Autodesk Fusion 360 part; units mm, degrees
note: some values were not read from the file. Chosen so that the rebuilt part matches the saved one: which face or edge a step refers to. Set by a fixed rule: which sketch regions a step uses.
(part 2 of 2)
extrude "Extrude26" cut sketch "Enclosure_upper" along normal blind 2 from surface at -3 contours L33 L34 L35 L36 bodies 2
extrude "Extrude27" add sketch "Enclosure_main" along normal blind 5 contours A4 | A6 | A8 | A9 | A12 | A13 | A14 | A18 | A19 | A22 | A23 bodies 1
sketch "bkac_plate" plane through (0, 0, -3) normal (0, 0, -1) x (-1, 0, 0)
  line L0 (-20, 60) -> (-210, 60)
  line L1 (-210, 60) -> (-210, -3)
  line L2 (-210, -3) -> (-20, -3)
  line L3 (-20, -3) -> (-20, 60)
  line L4 (-56.5, 6.25) -> (-39.5, 6.25)
  line L5 (-39.5, 6.25) -> (-39.5, 1.25)
  line L6 (-39.5, 1.25) -> (-56.5, 1.25)
  line L7 (-56.5, 1.25) -> (-56.5, 6.25)
  line L8 (3, -3) -> (3, 60)
  line L9 (-133.8, 16.5) -> (-117.5, 16.5)
  line L10 (-117.5, 16.5) -> (-117.5, 3)
  line L11 (-117.5, 3) -> (-133.8, 3)
  line L12 (-133.8, 3) -> (-133.8, 16.5)
  line L13 (0, 0) -> (-230, 0)
  circle A0 centre (-139.55, 11) radius 2
  circle A1 centre (-111.75, 11) radius 2
  circle A2 centre (-198.8, 12) radius 8
  circle A3 centre (-198.8, 37) radius 6
  line L14 (-206.05, 19.25) -> (-191.55, 19.25)
  line L15 (-191.55, 19.25) -> (-191.55, 4.75)
  line L16 (-191.55, 4.75) -> (-206.05, 4.75)
  line L17 (-206.05, 4.75) -> (-206.05, 19.25)
  line L18 (-206.05, 12) -> (-191.55, 12) construction
  line L19 (-198.8, 19.25) -> (-198.8, 4.75) construction
  line L20 (-204.25, 42.45) -> (-193.35, 42.45)
  line L21 (-193.35, 42.45) -> (-193.35, 31.55)
  line L22 (-193.35, 31.55) -> (-204.25, 31.55)
  line L23 (-204.25, 31.55) -> (-204.25, 42.45)
  line L24 (-204.25, 37) -> (-193.35, 37) construction
  line L25 (-198.8, 42.45) -> (-198.8, 31.55) construction
  circle A4 centre (-183.8, 25) radius 3.25
  point P0 (0, -20)
  dimension "d451" = 17
  dimension "d452" = 5
  dimension "d453" = 51
  dimension "d454" = 4.25
  dimension "d459" = 16.3
  dimension "d460" = 13.5
  dimension "d461" = 3
  dimension "d462" = 4
  dimension "d463" = 5.75
  dimension "d464" = 4
  dimension "d465" = 5.75
  dimension "d467" = 61
  dimension "d468" = 16
  dimension "d472" = 15
  dimension "d473" = 65
  dimension "d474" = 12
  dimension "d475" = 25
  dimension "d476" = 14.5
  dimension "d477" = 14.5
  dimension "d478" = 10.9
  dimension "d479" = 10.9
  dimension "d480" = 11
  dimension "d481" = 11
  dimension "d521" = 6.5
  dimension "d522" = 15
  dimension "d523" = 25
  measures "d452" distance of P0
  measures "d453" distance of P0 L8
  measures "d454" distance of L2 P0
  measures "d461" distance of L11 L13
  measures "d462" diameter of A0
  measures "d464" diameter of A1
  measures "d467" distance of P0
  measures "d468" diameter of A2
  measures "d472" distance of L2
  measures "d473" distance of L12
  measures "d474" diameter of A3
  measures "d475" distance of L13.start
  measures "d521" diameter of A4
  measures "d522" distance of L13.start
extrude "Extrude29" cut sketch "bkac_plate" against normal up to surface (3 mm away) contours L4 L5 L6 L7 | L9 L10 L11 L12 | A0 | A1 | A2 L14 L15 L16 L17 | A2 L14 | A2 L16 | A3 L20 L21 L22 L23 | A3 L20 | A3 L22 | A4 bodies 1
fillet "Fillet10" radius 2 8 edges at (39.5, 3.75, -3) (48, 6.25, -3) (56.5, 3.75, -3) (48, 1.25, -3) (133.8, 9.75, -3) (125.65, 16.5, -3) (117.5, 9.75, -3) (125.65, 3, -3) on bodies 1
chamfer "Chamfer3" distance 1.5 angle 45 2 edges at (141.4147, 11.7232, -3) (113.6147, 11.7232, -3) on bodies 1
named bodies: "enclosure_lower", "enclosure_upper", "OLED_holder"
